Autodesk Inventor part; units mm, degrees
(part 2 of 2)
sketch "Sketch120" plane through (0, 0, 52) normal (0, 0, -1) x (-1, 0, 0)
  line L0 (-5.5, 48.7965) -> (-5.5, 49.7965) projected
  line L1 (-5.5, 47.9965) -> (-5.5, 48.7965) projected
  line L2 (-5.5, 47.9965) -> (-5.5, 45.9965) projected
  line L3 (-5.5, 45.9965) -> (-5.5, 19.7965) projected
  line L4 (-5.5, 19.7965) -> (-5.5, 45.9965) projected
  line L5 (-5.5, 45.9965) -> (-5.5, 47.9965) projected
  line L6 (-5.5, 48.7965) -> (-5.5, 47.9965) projected
  line L7 (-5.5, 49.7965) -> (-5.5, 48.7965) projected
  line L8 (-5.5, -48.7965) -> (-5.5, -49.7965) projected
  line L9 (-5.5, -47.9965) -> (-5.5, -48.7965) projected
  line L10 (-5.5, -47.9965) -> (-5.5, -45.9965) projected
  line L11 (-5.5, -45.9965) -> (-5.5, -19.7965) projected
  line L12 (-5.5, -19.7965) -> (-5.5, -45.9965) projected
  line L13 (-5.5, -45.9965) -> (-5.5, -47.9965) projected
  line L14 (-5.5, -48.7965) -> (-5.5, -47.9965) projected
  line L15 (-5.5, -49.7965) -> (-5.5, -48.7965) projected
  line L16 (-6, 5.3855) -> (-6, 46.7965) projected
  line L17 (-6, -46.7965) -> (-6, -5.3855) projected
  line L18 (-6, 46.7965) -> (-3.5, 46.7965)
  line L19 (-3.5, 46.7965) -> (-3.5, 17.7965)
  line L20 (-3.5, 17.7965) -> (-6, 17.7965)
  line L21 (-6, 17.7965) -> (-6, 46.7965)
  line L22 (-6, -46.7965) -> (-3.5, -46.7965)
  line L23 (-3.5, -46.7965) -> (-3.5, -17.7965)
  line L24 (-3.5, -17.7965) -> (-6, -17.7965)
  line L25 (-6, -17.7965) -> (-6, -46.7965)
  point P0 (0, 0)
  dimension "d491" = 2
  dimension "d492" = 2
  dimension "d493" = 2
  constraints: 16 end point, 4 parallel, 2 horizontal, 2 perpendicular, 1 vertical alignment
  measures "d491" distance between parallel lines of L19 L3
  measures "d492" distance from line of L20 L3.end
  measures "d493" distance from line of L24 L11.end
extrude "Extrusion103" add sketch "Sketch120" along normal blind 2
sketch "Sketch123" plane through (9, -49.7965, 50) normal (1, 0, 0) x (0, 0, -1)
  line L0 (-2, 99.5929) -> (-5, 99.5929)
  line L1 (-5, 99.5929) -> (-5, 69.5929)
  line L2 (-5, 69.5929) -> (-2, 69.5929)
  line L3 (-2, 69.5929) -> (-2, 99.5929)
  line L4 (-3, 69.5929) -> (-32, 69.5929) projected
  line L5 (-3, 98.5929) -> (-3, 97.7929) projected
  line L6 (-3, 69.5929) -> (-35, 69.5929) projected
  line L7 (-19, 69.5929) -> (-19, 30)
  line L8 (-35, 30) -> (-3, 30) projected
  line L9 (0, 49.7965) -> (-70, 49.7965) projected
  line L10 (-2, 0) -> (-5, 0)
  line L11 (-5, 0) -> (-5, 30)
  line L12 (-5, 30) -> (-2, 30)
  line L13 (-2, 30) -> (-2, 0)
  line L14 (-36, 99.5929) -> (-33, 99.5929)
  line L15 (-33, 99.5929) -> (-33, 69.5929)
  line L16 (-33, 69.5929) -> (-36, 69.5929)
  line L17 (-36, 69.5929) -> (-36, 99.5929)
  line L18 (-33, 0) -> (-33, 30)
  line L19 (-36, 30) -> (-36, 0)
  line L20 (-33, 30) -> (-36, 30)
  line L21 (-36, 0) -> (-33, 0)
  point P0 (50, 49.7965)
  dimension "d494" = 2
  constraints: 34 end point, 12 symmetric about line, 2 midpoint, 2 parallel, 1 horizontal, 1 perpendicular, 1 point on line
  measures "d494" distance between parallel lines of L1 L5
extrude "Extrusion105" add sketch "Sketch123" against normal blind 1
sketch "Sketch125" plane through (5.5, -49.7965, 50) normal (1, 0, 0) x (0, 0, -1)
  line L0 (-36, 99.5929) -> (-2, 99.5929) projected
  line L1 (-35, 98.5929) -> (-36, 99.5929) projected
  line L2 (-35, 97.7929) -> (-35, 98.5929) projected
  line L3 (-35, 97.7929) -> (-35.6, 97.7929) projected
  line L4 (-35.6, 97.7929) -> (-35.6, 95.7929) projected
  line L5 (-35.6, 95.7929) -> (-35, 69.5929) projected
  line L6 (-3, 69.5929) -> (-35, 69.5929) projected
  line L7 (-3, 69.5929) -> (-2.4, 95.7929) projected
  line L8 (-2.4, 95.7929) -> (-2.4, 97.7929) projected
  line L9 (-2.4, 97.7929) -> (-3, 97.7929) projected
  line L10 (-3, 98.5929) -> (-3, 97.7929) projected
  line L11 (-2, 99.5929) -> (-3, 98.5929) projected
  line L12 (-2, 0) -> (-36, 0) projected
  line L13 (-3, 1) -> (-2, 0) projected
  line L14 (-3, 1.8) -> (-3, 1) projected
  line L15 (-3, 1.8) -> (-2.4, 1.8) projected
  line L16 (-2.4, 1.8) -> (-2.4, 3.8) projected
  line L17 (-2.4, 3.8) -> (-3, 30) projected
  line L18 (-35, 30) -> (-3, 30) projected
  line L19 (-35, 30) -> (-35.6, 3.8) projected
  line L20 (-35.6, 3.8) -> (-35.6, 1.8) projected
  line L21 (-35.6, 1.8) -> (-35, 1.8) projected
  line L22 (-35, 1) -> (-35, 1.8) projected
  line L23 (-36, 0) -> (-35, 1) projected
  point P0 (50, 49.7965)
extrude "Extrusion106" cut sketch "Sketch125" against normal blind 1
body "Solid2"
